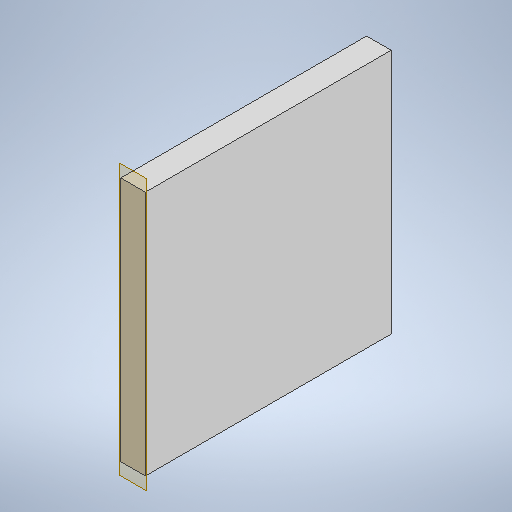
# Autodesk Inventor part: hole2025
Saved by Autodesk Inventor 2026 (Build 300175050, 175E)
## iProperties
Created: 2025-09-06
Part Number: hole2025
Material: Generic
Document SubType Name: Modeling
Designer: TiffanyHayden
Density: 1 g/cm^3
Appearance: Default
Author: TiffanyHayden
Autodesk Inventor part; units mm, degrees
ref_plane "YZ Plane" through (0, 0, 0) normal (1, 0, 0) x (0, 1, 0)
ref_plane "XZ Plane" through (0, 0, 0) normal (0, 1, 0) x (-1, 0, 0)
ref_plane "Left Side" through (0, 0, 127) normal (0, 0, 1) x (1, 0, 0)
sketch "Sketch1" plane through (0, 0, 0) normal (1, 0, 0) x (0, 1, 0)
  line L0 (-127, 127) -> (127, 127)
  line L1 (127, 127) -> (127, -127)
  line L2 (127, -127) -> (-127, -127)
  line L3 (-127, -127) -> (-127, 127)
  line L4 (-127, 127) -> (127, -127) construction
  line L5 (127, 127) -> (-127, -127) construction
  point P0 (0, 0)
  dimension "d0" = 254
  dimension "d1" = 254
  constraints: 12 end point, 2 midpoint, 2 parallel, 1 horizontal, 1 perpendicular
  measures "d0" distance of L1.end L2.end
  measures "d1" distance of L0.end L1.end
extrude "Plate" add sketch "Sketch1" against normal blind 25.4
body "Solid1"
